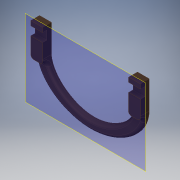
# Autodesk Inventor part: ArmsBottomLongHalf
Saved by Autodesk Inventor 2017 (Build 210142000, 142)
## iProperties
Created: 2017-01-25
Part Number: ArmsBottomLongHalf
Material: Bronze, Soft Tin
Document SubType Name: Modeling
Designer: aribu
Density: 8.874 g/cm^3
Appearance: Bronze - Satin
Author: aribu
Autodesk Inventor part; units mm, degrees
ref_plane "YZ Plane" through (0, 0, 0) normal (1, 0, 0) x (0, 1, 0)
ref_plane "XZ Plane" through (0, 0, 0) normal (0, 1, 0) x (-1, 0, 0)
ref_plane "XY Plane" through (0, 0, 0) normal (0, 0, 1) x (1, 0, 0)
sketch "Sketch1" plane through (0, 0, 0) normal (0, 0, 1) x (1, 0, 0)
  line L0 (-27.4851, 19.0486) -> (-14.7851, 19.0486)
  line L1 (-14.7851, 19.0486) -> (-14.7851, -10.9514)
  line L2 (-27.4851, -10.9514) -> (-27.4851, 19.0486)
  spline S0 degree 3 poles (-27.4851, -10.9514) (-26.3032, -37.8438) (3.0299, -55.8593) (31.5149, -55.9514) knots 0 0 0 0 1 1 1 1
  spline S1 degree 3 poles (-14.7851, -10.9514) (-12.7754, -30.3317) (10.5153, -46.1534) (31.5149, -45.9621) knots 0 0 0 0 1 1 1 1
  line L3 (90.5149, 19.0486) -> (77.8149, 19.0486)
  line L4 (77.8149, 19.0486) -> (77.8149, -10.9514)
  line L5 (90.5149, -10.9514) -> (90.5149, 19.0486)
  spline S2 degree 3 poles (90.5149, -10.9514) (89.3325, -37.8433) (60.0002, -55.859) (31.5149, -55.9514) knots 0 0 0 0 1 1 1 1
  spline S3 degree 3 poles (77.8149, -10.9514) (75.8052, -30.3316) (52.5145, -46.1533) (31.5149, -45.9621) knots 0 0 0 0 1 1 1 1
  point P0 (0, 0)
  point P1 (-18.8189, -33.5357)
  point P2 (2.4622, -49.6218)
  point P3 (-7.3212, -27.7766)
  point P4 (9.9678, -40.9715)
  point P5 (63.0299, 0)
  point P6 (81.8486, -33.5353)
  point P7 (60.5678, -49.6214)
  point P8 (70.351, -27.7766)
  point P9 (53.062, -40.9714)
  dimension "d0" = 12.7
  dimension "d2" = 30
  dimension "d3" = 30
  dimension "d27" = 75
  dimension "d28" = 59
  dimension "d84" = 65.0107
  constraints: 12 end point, 1 horizontal, 1 parallel, 1 perpendicular, 16 other
  measures "d0" distance of L0.start L0.end
  measures "d2" distance of L0.end L1.end
  measures "d3" distance of L2.start L0.start
  measures "d27" vertical distance of point (31.515, -55.951) L0.start
  measures "d28" horizontal distance of point (31.515, -45.962) L0.start
  measures "d84" distance from line of L0 point (31.515, -45.962)
extrude "Extrusion1" add sketch "Sketch1" along normal blind 19.05
sketch "Sketch5" plane through (90.5149, -10.9514, 0) normal (1, 0, 0) x (0, 0, -1)
  line L0 (-14.225, 25.175) -> (-4.825, 25.175)
  line L1 (-4.825, 25.175) -> (-4.825, 15.775)
  line L2 (-4.825, 15.775) -> (-14.225, 15.775)
  line L3 (-14.225, 15.775) -> (-14.225, 25.175)
  line L4 (0, 30) -> (-19.05, 30)
  line L5 (0, 10.95) -> (-19.05, 10.95)
  line L6 (-19.05, 10.95) -> (-19.05, 30)
  line L7 (0, 30) -> (0, 10.95)
  line L8 (0, 30) -> (-19.05, 30)
  point P0 (0, 0.657)
  dimension "d62" = 4.825
  dimension "d63" = 4.825
  dimension "d64" = 4.825
  dimension "d65" = 4.825
  dimension "d75" = 0
  dimension "d76" = 9.4
  dimension "d77" = 9.4
  constraints: 18 end point, 2 parallel, 1 horizontal, 1 perpendicular
  measures "d62" distance between parallel lines of L4 L0
  measures "d63" distance between parallel lines of L5 L2
  measures "d64" distance between parallel lines of L6 L3
  measures "d65" distance between parallel lines of L7 L1
  measures "d75" distance between parallel lines of L8 L4
  measures "d76" distance of L0.start L0.end
  measures "d77" distance of L2.end L0.start
extrude "Extrusion5" cut sketch "Sketch5" against normal blind 177.8 contours L0 L1 L2 L3
sketch "Sketch7" plane through (90.5149, -10.9514, 0) normal (1, 0, 0) x (0, 0, -1)
  arc A0 (-4.7625, -9.525) -> (-14.2875, -9.525) centre (-9.525, -9.525) ccw
  line L0 (0, 30) -> (0, 0)
  line L1 (0, 0) -> (-19.05, 0)
  line L2 (-14.2875, -9.525) -> (-14.2875, -46.9526)
  line L3 (-14.2875, -46.9526) -> (-4.7625, -46.9526)
  line L4 (-4.7625, -46.9526) -> (-4.7625, -9.525)
  point P0 (0, 10.8159)
  dimension "d78" = 9.525
  dimension "d79" = 9.525
  dimension "d80" = 9.525
  constraints: 10 end point, 2 perpendicular, 2 point on circle, 1 centre point, 1 vertical
  measures "d78" diameter of A0
  measures "d79" distance from line of L0 A0.centre
  measures "d80" distance from line of A0.centre L1
extrude "Extrusion7" cut sketch "Sketch7" against normal blind 120
fillet "Fillet8" radius 3.175 12 edges at (76.8831, -15.714, 9.5607) (56.7537, -39.0499, 14.2875) (56.7537, -39.0499, 4.7625) (-13.8533, -15.714, 9.5607) (6.2762, -39.0499, 14.2875) (6.2762, -39.0499, 4.7625) (90.0009, -15.7139, 9.5247) (65.8583, -46.9344, 4.7625) (65.8583, -46.9344, 14.2875) (-26.9712, -15.7139, 9.5247) (-2.8287, -46.9346, 4.7625) (-2.8287, -46.9346, 14.2875)
ref_plane "Work Plane1" through (0, 0, 9.525) normal (0, 0, -1) x (-1, 0, 0)
split "Split1" plane through (0, 0, 9.525) removes the side toward (0, 0, 1)
body "Solid1"
